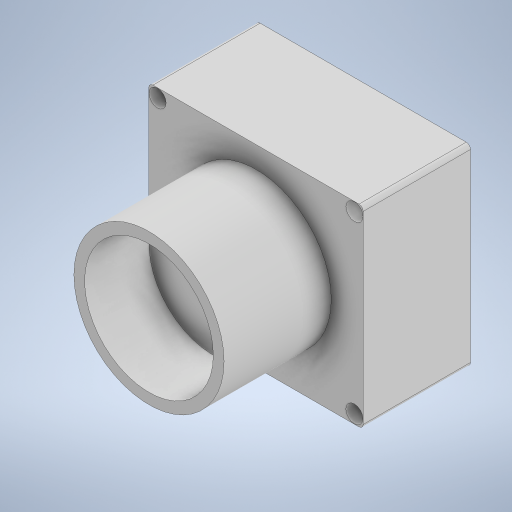
# Autodesk Inventor part: dinamica T1
Saved by Autodesk Inventor 2024 (Build 280153000, 153)
## iProperties
Created: 2024-02-05
Part Number: dinamica T1
Material: Genérico
Document SubType Name: Modeling
Designer: fenyc
Density: 1 g/cm^3
Appearance: Valor por defecto
Author: fenyc
Autodesk Inventor part; units mm, degrees
ref_plane "YZ Plane" through (0, 0, 0) normal (1, 0, 0) x (0, 1, 0)
ref_plane "XZ Plane" through (0, 0, 0) normal (0, 1, 0) x (-1, 0, 0)
ref_plane "XY Plane" through (0, 0, 0) normal (0, 0, 1) x (1, 0, 0)
sketch "Boceto1" plane through (0, 0, 0) normal (0, 0, 1) x (1, 0, 0)
  line L0 (2, 0) -> (98, 0)
  line L1 (100, 2) -> (100, 88)
  line L2 (98.0371, 89.9629) -> (1.9629, 89.9629)
  line L3 (0, 88) -> (0, 2)
  arc A0 (1.9629, 89.9629) -> (0, 88) centre (1.9629, 88) ccw
  arc A1 (100, 88) -> (98.0371, 89.9629) centre (98.0371, 88) ccw
  arc A2 (0, 2) -> (2, 0) centre (2, 2) ccw
  arc A3 (98, 0) -> (100, 2) centre (98, 2) ccw
  circle A4 centre (4, 85.9629) radius 4
  circle A5 centre (96, 85.9629) radius 4
  circle A6 centre (4, 4) radius 4
  circle A7 centre (96, 4) radius 4
  point P0 (0, 0)
  point P1 (100, 89.9629)
  point P2 (100, 0)
  point P3 (0, 89.9629)
  dimension "d0" = 100
  dimension "d6" = 8
  dimension "d7" = 8
  dimension "d8" = 8
  dimension "d9" = 8
  constraints: 15 tangent, 8 centre point, 8 end point, 8 point on circle, 8 point on line, 2 parallel, 1 horizontal, 1 perpendicular
  measures "d0" distance of point (0, 89.963) point (100, 89.963)
  measures "d6" diameter of A4
  measures "d7" diameter of A5
  measures "d8" diameter of A6
  measures "d9" diameter of A7
extrude "Extrusión1" add sketch "Boceto1" along normal blind 50
sketch "Boceto2" plane through (0, 0, 50) normal (0, 0, 1) x (1, 0, 0)
  circle A0 centre (4.1038, 85.8268) radius 4
  circle A1 centre (95.7307, 85.8268) radius 4
  point P0 (0, 0)
  dimension "d12" = 8
  dimension "d13" = 8
  constraints: 2 centre point
  measures "d12" diameter of A0
  measures "d13" diameter of A1
hole "Agujero1" at (4.1038, 85.8268, 50) direction (0, 0, -1) diameter 8 end through all
sketch "Boceto3" plane through (0, 0, 50) normal (0, 0, 1) x (1, 0, 0)
  circle A0 centre (95.9335, 85.8863) radius 4
  point P0 (0, 0)
  dimension "d21" = 8
  constraints: 1 centre point
  measures "d21" diameter of A0
hole "Agujero2" at (95.9335, 85.8863, 50) direction (0, 0, -1) diameter 8 end through all
sketch "Boceto4" plane through (0, 0, 50) normal (0, 0, 1) x (1, 0, 0)
  circle A0 centre (95.8814, 4.2134) radius 4
  point P0 (0, 0)
  dimension "d29" = 8
  constraints: 1 centre point
  measures "d29" diameter of A0
hole "Agujero3" at (95.8814, 4.2134, 50) direction (0, 0, -1) diameter 8 end through all
sketch "Boceto5" plane through (0, 0, 50) normal (0, 0, 1) x (1, 0, 0)
  circle A0 centre (4.0599, 4.0663) radius 4
  point P0 (0, 0)
  dimension "d37" = 8
  constraints: 1 centre point
  measures "d37" diameter of A0
hole "Agujero4" at (4.0599, 4.0663, 50) direction (0, 0, -1) diameter 8 end through all
sketch "Boceto6" plane through (0, 0, 50) normal (0, 0, 1) x (1, 0, 0)
  circle A0 centre (50.1065, 44.9629) radius 35
  line L0 (98.0371, 89.9629) -> (1.9629, 89.9629) projected
  line L1 (2, 0) -> (98, 0) projected
  circle A1 centre (50.1065, 44.9629) radius 30
  point P0 (0, 0)
  point P1 (50, 89.9629)
  point P2 (50, 0)
  dimension "d45" = 70
  dimension "d48" = 60
  constraints: 2 centre point, 2 midpoint, 1 coincident
  measures "d45" diameter of A0
  measures "d48" diameter of A1
extrude "Extrusión2" add sketch "Boceto6" along normal blind 50
sketch "Boceto7" plane through (50.1065, 44.9629, 50) normal (0, 0, 1) x (1, 0, 0)
  circle A0 centre (0, 0) radius 30
  point P0 (-50.1065, -44.9629)
  dimension "d51" = 60
  constraints: 1 centre point
  measures "d51" diameter of A0
extrude "Extrusión3" add sketch "Boceto7" along normal blind 20
